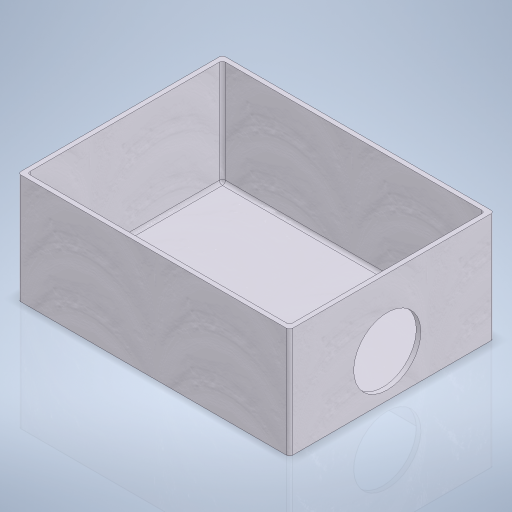
# Autodesk Inventor part: 102 part 1
Saved by Autodesk Inventor 2024 (Build 280153000, 153)
## iProperties
Created: 2024-07-24
Part Number: 102 part 1
Material: Aluminum 6061, geschweißt
Document SubType Name: Modeling
Designer: ffogue
Density: 2.7 g/cm^3
Appearance: Schweißnaht - Aluminum
Author: ffogue
Autodesk Inventor part; units mm, degrees
ref_plane "YZ Plane" through (0, 0, 0) normal (1, 0, 0) x (0, 1, 0)
ref_plane "XZ Plane" through (0, 0, 0) normal (0, 1, 0) x (-1, 0, 0)
ref_plane "XY Plane" through (0, 0, 0) normal (0, 0, 1) x (1, 0, 0)
sketch "Skizze2" plane through (0, 0, 0) normal (0, 0, 1) x (1, 0, 0)
  line L0 (-44.5, 0) -> (44.5, 0)
  line L1 (44.5, 0) -> (44.5, 67)
  line L2 (44.5, 67) -> (-44.5, 67)
  line L3 (-44.5, 67) -> (-44.5, 0)
  point P0 (0, 0)
  point P1 (0, 0)
  dimension "d0" = 89
  dimension "d1" = 67
  constraints: 8 end point, 2 parallel, 1 coincident, 1 horizontal, 1 midpoint, 1 perpendicular
  measures "d0" distance of L1.end L2.end
  measures "d1" distance between parallel lines of L0 L2
extrude "Extrusion1" add sketch "Skizze2" along normal blind 36
shell "Wandung1" thickness 1.5 removed faces 1 at (-14.8333, 44.6667, 36)
sketch "Skizze3" plane through (44.5, 0, 0) normal (1, 0, 0) x (0, 0, -1)
  circle A0 centre (-14, 32) radius 11
  line L0 (0, 0) -> (0, 67) projected
  line L1 (0, 67) -> (-36, 67) projected
  dimension "d5" = 22
  dimension "d6" = 14
  dimension "d7" = 35
  constraints: 1 centre point
  measures "d5" diameter of A0
  measures "d6" distance from line of L0 A0.centre
  measures "d7" distance from line of L1 A0.centre
extrude "Extrusion2" cut sketch "Skizze3" against normal up to surface (1.5 mm away)
fillet "Rundung1" radius 1 12 edges at (44.5, 67, 18) (44.5, 0, 18) (-44.5, 0, 18) (-44.5, 67, 18) (-43, 65.5, 18.75) (43, 65.5, 18.75) (43, 1.5, 18.75) (-43, 1.5, 18.75) (-43, 33.5, 1.5) (0, 1.5, 1.5) (43, 33.5, 1.5) (0, 65.5, 1.5)
